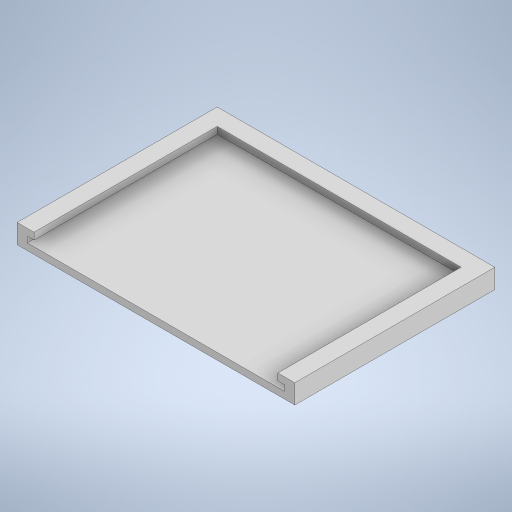
# Autodesk Inventor part: podstawka_na_pcb
Saved by Autodesk Inventor 2023 (Build 270158000, 158)
## iProperties
Created: 2024-04-25
Part Number: podstawka_na_pcb
Material: Ogólny
Document SubType Name: Modeling
Designer: Kamil
Density: 1 g/cm^3
Appearance: Domyślna
Author: Kamil
Autodesk Inventor part; units mm, degrees
ref_plane "YZ Plane" through (0, 0, 0) normal (1, 0, 0) x (0, 1, 0)
ref_plane "XZ Plane" through (0, 0, 0) normal (0, 1, 0) x (-1, 0, 0)
ref_plane "XY Plane" through (0, 0, 0) normal (0, 0, 1) x (1, 0, 0)
sketch "Szkic1" plane through (0, 0, 0) normal (0, 1, 0) x (-1, 0, 0)
  line L0 (7, 46.073) -> (-75, 46.073)
  line L1 (-75, 46.073) -> (-75, -13)
  line L2 (-75, -13) -> (7, -13)
  line L3 (7, -13) -> (7, 46.073)
  point P0 (0, 0)
  dimension "d0" = 82
  dimension "d1" = 59.073
  constraints: 8 end point, 2 parallel, 1 horizontal, 1 perpendicular
  measures "d0" distance of L2.end L1.end
  measures "d1" distance of L2.end L0.start
extrude "Wyciągnięcie proste1" add sketch "Szkic1" along normal blind 2
sketch "Szkic2" plane through (0, 2, 0) normal (0, 1, 0) x (1, 0, 0)
  line L0 (75, -46.073) -> (75, 13) projected
  line L1 (75, 13) -> (-7, 13) projected
  line L2 (-7, 13) -> (-7, -46.073) projected
  line L3 (-7, -46.073) -> (75, -46.073) projected
  line L4 (-4, 10) -> (72, 10)
  line L5 (72, 10) -> (72, -43.073)
  line L6 (72, -43.073) -> (-4, -43.073)
  line L7 (-4, -43.073) -> (-4, 10)
  line L8 (-4, -43.073) -> (-4, -46.073)
  line L9 (72, -43.073) -> (72, -46.073)
  line L10 (-7, -46.073) -> (75, -46.073) projected
  point P0 (0, 0)
  dimension "d4" = 3
  constraints: 12 end point, 2 perpendicular, 2 point on line, 3 other
  measures "d4" distance between parallel lines of L1 L4
extrude "Wyciągnięcie proste2" add sketch "Szkic2" along normal blind 1.7 contours L3 L9 L5 L4 L7 L8 L2 L1 L0
sketch "Szkic3" plane through (0, 3.7, 0) normal (0, 1, 0) x (1, 0, 0)
  line L0 (75, 13) -> (-7, 13) projected
  line L1 (-7, 13) -> (-7, -46.073) projected
  line L2 (-7, -46.073) -> (-4, -46.073) projected
  line L3 (72, -46.073) -> (75, -46.073) projected
  line L4 (75, -46.073) -> (75, 13) projected
  line L5 (72, -46.073) -> (72, 10) projected
  line L6 (72, 10) -> (-4, 10) projected
  line L7 (-4, 10) -> (-4, -46.073) projected
  line L8 (-4, -46.073) -> (72, -46.073) projected
  line L9 (-2, 8) -> (70, 8)
  line L10 (70, 8) -> (70, -44.073)
  line L11 (70, -44.073) -> (-2, -44.073)
  line L12 (-2, -44.073) -> (-2, 8)
  line L13 (-2, -44.073) -> (-2, -46.073)
  line L14 (-7, -46.073) -> (75, -46.073) projected
  line L15 (70, -44.073) -> (70, -46.073)
  point P0 (0, 0)
  dimension "d7" = 2
  constraints: 12 end point, 2 point on line, 1 perpendicular, 1 vertical, 3 other
  measures "d7" distance between parallel lines of L6 L9
extrude "Wyciągnięcie proste3" add sketch "Szkic3" along normal blind 2 contours L4 L3 L5 L6 L7 L2 L1 L0 | L8 L15 L10 L9 L12 L13 L7 L6 L5
